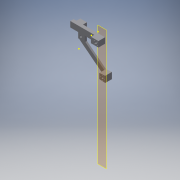
# Autodesk Inventor part: support
Saved by Autodesk Inventor 2016 (Build 200138000, 138)
## iProperties
Created: 2015-12-09
Part Number: support
Material: Generic
Document SubType Name: Modeling
Designer: Julia
Density: 1 g/cm^3
Appearance: Default
Author: Julia
Autodesk Inventor part; units mm, degrees
ref_plane "YZ Plane" through (0, 0, 0) normal (1, 0, 0) x (0, 1, 0)
ref_plane "XZ Plane" through (0, 0, 0) normal (0, 1, 0) x (-1, 0, 0)
ref_plane "XY Plane" through (0, 0, 0) normal (0, 0, 1) x (1, 0, 0)
ref_plane "Work Plane1" through (0, 0, 0) normal (0, 0, 1) x (1, 0, 0)
sketch "Sketch1" plane through (0, 0, 0) normal (0, 0, 1) x (1, 0, 0)
  line L0 (-1.8708, -26.7127) -> (26.5352, -26.7127)
  line L1 (26.5352, -26.7127) -> (26.5352, -5.4733)
  line L2 (26.5352, -5.4733) -> (-1.8708, -5.4733)
  line L3 (-1.8708, -5.4733) -> (-1.8708, -26.7127)
  point P0 (0, 0)
  constraints: 8 end point, 2 parallel, 1 horizontal, 1 perpendicular
extrude "Extrusion1" add sketch "Sketch1" along normal blind 25.4
sketch "Sketch2" plane through (-1.8708, -26.7127, 0) normal (-1, 0, 0) x (0, 0, 1)
  line L0 (0, 0) -> (25.4, 0) projected
  line L1 (0, 21.2393) -> (25.4, 21.2393) projected
  line L2 (12.7, 0) -> (0, 0)
  line L3 (0, 0) -> (0, 21.2393)
  line L4 (0, 21.2393) -> (12.7, 21.2393)
  line L5 (12.7, 21.2393) -> (12.7, 0)
  point P0 (0, 26.7127)
  constraints: 8 end point, 2 parallel, 1 horizontal, 1 midpoint, 1 perpendicular
extrude "Extrusion2" add sketch "Sketch2" along normal blind 91.44
sketch "Sketch3" plane through (0, 0, 0) normal (0, 0, -1) x (-1, 0, 0)
  line L0 (93.3108, -5.4733) -> (93.3108, -26.7127) projected
  line L1 (93.3108, -26.7127) -> (-26.5352, -26.7127) projected
  line L2 (93.3108, -16.093) -> (67.944, -16.093)
  line L3 (67.944, -16.093) -> (67.944, -26.7127)
  line L4 (67.944, -26.7127) -> (93.3108, -26.7127)
  line L5 (93.3108, -26.7127) -> (93.3108, -16.093)
  point P0 (0, 0)
  constraints: 8 end point, 2 parallel, 1 horizontal, 1 midpoint, 1 perpendicular, 1 point on line
extrude "Extrusion3" add sketch "Sketch3" along normal blind 25.4
sketch "Sketch4" plane through (-1.8708, -26.7127, 25.4) normal (0, -1, 0) x (1, 0, 0)
  line L0 (-91.44, -12.7) -> (-91.44, -50.8) projected
  line L1 (-66.0732, -25.4) -> (-66.0732, -50.8) projected
  line L2 (-91.44, -50.8) -> (-66.0732, -50.8)
  line L3 (-66.0732, -50.8) -> (-66.0732, -42.7329)
  line L4 (-66.0732, -42.7329) -> (-91.44, -42.7329)
  line L5 (-91.44, -42.7329) -> (-91.44, -50.8)
  point P0 (1.8708, -25.4)
  constraints: 8 end point, 2 parallel, 1 horizontal, 1 perpendicular, 1 point on line
extrude "Extrusion4" add sketch "Sketch4" along normal blind 50.8
sketch "Sketch5" plane through (0, 0, 25.4) normal (0, 0, 1) x (1, 0, 0)
  point P0 (0, 0)
sketch "Sketch6" plane through (0, 0, 0) normal (0, 0, 1) x (1, 0, 0)
  point P0 (0, 0)
sketch "Sketch7" plane through (0, 0, 0) normal (0, 0, -1) x (-1, 0, 0)
  circle A0 centre (-10.3431, -10.3431) radius 1.85 projected
  circle A1 centre (-8, -16) radius 1.85 projected
  circle A2 centre (-10.3431, -21.6569) radius 1.85 projected
  circle A3 centre (-16, -24) radius 1.85 projected
  circle A4 centre (-16, -8) radius 1.85 projected
  circle A5 centre (-21.6569, -10.3431) radius 1.85 projected
  circle A6 centre (-24, -16) radius 1.85 projected
  circle A7 centre (-21.6569, -21.6569) radius 1.85 projected
  circle A8 centre (-16, -16) radius 4 projected
  circle A9 centre (-16, -16) radius 4
  point P0 (0, 0)
  constraints: 1 centre point, 1 coincident, 1 concentric
extrude "Extrusion5" cut sketch "Sketch7" against normal blind 31.75 contours A8
sketch "Sketch8" plane through (0, 0, 0) normal (0, 0, -1) x (-1, 0, 0)
  circle A0 centre (-10.3431, -10.3431) radius 1.85 projected
  circle A1 centre (-10.3431, -10.3431) radius 1.85
  point P0 (0, 0)
  constraints: 1 centre point, 1 coincident, 1 concentric
extrude "Extrusion6" cut sketch "Sketch8" against normal blind 30.1625
sketch "Sketch9" plane through (0, 0, 0) normal (0, 0, -1) x (-1, 0, 0)
  circle A0 centre (-21.6569, -21.6569) radius 1.85 projected
  circle A1 centre (-10.3431, -21.6569) radius 1.85 projected
  circle A2 centre (-21.6569, -10.3431) radius 1.85 projected
  circle A3 centre (-21.6569, -10.3431) radius 1.85
  circle A4 centre (-10.3431, -21.6569) radius 1.85
  circle A5 centre (-21.6569, -21.6569) radius 1.85
  point P0 (0, 0)
  constraints: 3 centre point, 3 coincident, 3 concentric
extrude "Extrusion7" cut sketch "Sketch9" against normal blind 42.8625
sketch "Sketch10" plane through (-93.3108, -26.7127, -17.3329) normal (0, 0, 1) x (1, 0, 0)
  circle A0 centre (9.3305, -39.9903) radius 4
  circle A1 centre (9.3305, -39.9903) radius 4 projected
  point P0 (93.3108, 26.7127)
  constraints: 1 centre point, 1 concentric
extrude "Extrusion8" cut sketch "Sketch10" against normal blind 38.1
sketch "Sketch11" plane through (0, 0, -25.4) normal (0, 0, -1) x (-1, 0, 0)
  line L0 (67.944, -77.5127) -> (93.3108, -77.5127) projected
  line L1 (93.3108, -77.5127) -> (-4.4164, -154.1391)
  line L2 (-4.4164, -154.1391) -> (-27.0497, -155.9193)
  line L3 (-27.0497, -155.9193) -> (-27.0497, -132.2688)
  line L4 (-27.0497, -132.2688) -> (-4.1962, -134.0767)
  line L5 (-4.1962, -134.0767) -> (67.944, -77.5127)
  point P0 (0, 0)
  constraints: 10 end point, 1 parallel, 1 perpendicular
extrude "Extrusion9" add sketch "Sketch11" against normal blind 6.35
sketch "Sketch12" plane through (4.4164, -154.1391, -25.4) normal (-0.6170287, -0.7869406, 0) x (0.7869406, -0.6170287, 0)
  point P0 (-98.5837, 25.4)
sketch "Sketch13" plane through (0, 0, -19.05) normal (0, 0, 1) x (1, 0, 0)
  line L0 (-93.3108, -77.5127) -> (4.4164, -154.1391) projected
  line L1 (4.4164, -154.1391) -> (4.4164, -134.0593)
  line L2 (27.0497, -155.9193) -> (27.0497, -132.2688) projected
  line L3 (4.4164, -134.0593) -> (27.0497, -132.2688)
  line L4 (27.0497, -132.2688) -> (4.1962, -134.0767) projected
  line L5 (27.0497, -132.2688) -> (27.0497, -155.9193)
  line L6 (4.4164, -154.1391) -> (27.0497, -155.9193) projected
  line L7 (27.0497, -155.9193) -> (4.4164, -154.1391)
  line L8 (4.1962, -134.0767) -> (-67.944, -77.5127) projected
  line L9 (4.4164, -154.1391) -> (4.1962, -134.0767)
  point P0 (0, 0)
  constraints: 10 end point, 3 collinear, 1 vertical
extrude "Extrusion10" add sketch "Sketch13" along normal blind 19.05 contours L1 L3 L2 L6
sketch "Sketch14" plane through (0, 0, -25.4) normal (0, 0, -1) x (-1, 0, 0)
  circle A0 centre (-16.0005, -136) radius 1.85 projected
  circle A1 centre (-10.3436, -138.3431) radius 1.85 projected
  circle A2 centre (-8.0005, -144) radius 1.85 projected
  circle A3 centre (-10.3437, -149.6569) radius 1.85 projected
  circle A4 centre (-16.0005, -152) radius 1.85 projected
  circle A5 centre (-21.6574, -149.6568) radius 1.85 projected
  circle A6 centre (-24.0005, -143.9999) radius 1.85 projected
  circle A7 centre (-21.6573, -138.3431) radius 1.85 projected
  circle A8 centre (-16.0005, -144) radius 4 projected
  circle A9 centre (-16.0005, -144) radius 4
  circle A10 centre (-10.3437, -149.6569) radius 1.85
  circle A11 centre (-10.3436, -138.3431) radius 1.85
  circle A12 centre (-21.6573, -138.3431) radius 1.85
  circle A13 centre (-21.6574, -149.6568) radius 1.85
  point P0 (0, 0)
  constraints: 5 centre point, 5 coincident, 5 concentric
extrude "Extrusion11" cut sketch "Sketch14" against normal blind 65.0875 contours A0 | A2 | A4 | A6 | A8
body "Solid1"
